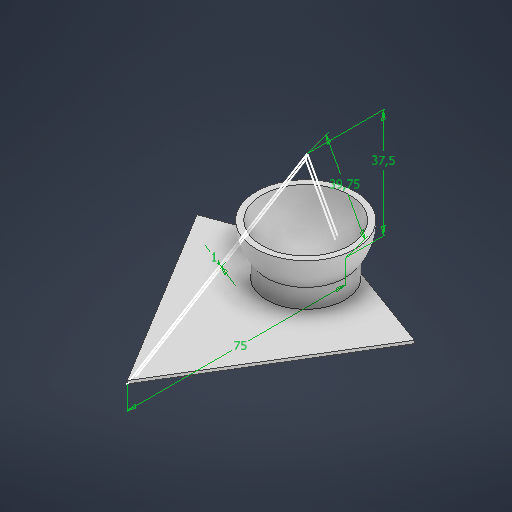
# Autodesk Inventor part: cabeza_1
Saved by Autodesk Inventor 2026.2 (Build 302298000, 298)
## iProperties
Created: 2026-05-21
Part Number: cabeza_1
Material: Generic
Document SubType Name: Modeling
Designer: juand
Density: 1 g/cm^3
Appearance: Default
Author: juand
Autodesk Inventor part; units mm, degrees
ref_plane "YZ Plane" through (0, 0, 0) normal (1, 0, 0) x (0, 1, 0)
ref_plane "XZ Plane" through (0, 0, 0) normal (0, 1, 0) x (-1, 0, 0)
ref_plane "XY Plane" through (0, 0, 0) normal (0, 0, 1) x (1, 0, 0)
sketch "Sketch1" plane through (0, 0, 0) normal (1, 0, 0) x (0, 1, 0)
  line L0 (0, 0) -> (0, 75)
  line L1 (0, 0) -> (37.5, 13.1838)
  line L2 (37.5, 13.1838) -> (0, 75)
  line L3 (0, 73.072) -> (36.006, 13.7185)
  line L4 (36.006, 13.7185) -> (0, 1.06)
  line L5 (36.006, 13.7185) -> (37.5, 13.1838)
  dimension "d0" = 75
  dimension "d1" = 37.5
  dimension "d2" = 39.75
  dimension "d3" = 1
  constraints: 12 end point, 2 point on line, 1 vertical, 1 other
  measures "d0" distance of L0.start L0.end
  measures "d1" horizontal distance of L1.end L0.start
  measures "d2" distance of L0.start L1.end
  measures "d3" distance between parallel lines of L2 L3
sketch "Sketch2" plane through (0, 0, 0) normal (0, 1, 0) x (-1, 0, 0)
  line L0 (0, 0) -> (-37.3077, 13.7185)
  line L1 (-37.3077, 13.7185) -> (0, 75)
  line L2 (0, 0) -> (0, 75) projected
  line L3 (0, 13.7185) -> (0, 1.06) projected
  line L4 (0, 13.7185) -> (-37.3077, 13.7185) construction
  line L5 (0, 1.0655) -> (-35.8211, 14.2374)
  line L6 (-35.8211, 14.2374) -> (0, 73.077)
  line L7 (0, 0) -> (37.3077, 13.7185)
  line L8 (37.3077, 13.7185) -> (0, 75)
  line L9 (0, 1.0655) -> (35.8211, 14.2374)
  line L10 (35.8211, 14.2374) -> (0, 73.077)
  line L11 (-35.8211, 14.2374) -> (-37.3077, 13.7185)
  line L12 (35.8211, 14.2374) -> (37.3077, 13.7185)
  dimension "d4" = 39.75
  dimension "d5" = 1
  constraints: 22 end point, 2 point on line, 2 symmetric about line, 1 perpendicular, 1 other
  measures "d4" distance of L0.start L0.end
  measures "d5" distance between parallel lines of L0 L5
extrude "Extrusion1" add sketch "Sketch2" along normal blind 1
sketch "Sketch6" plane through (0, 0, 0) normal (1, 0, 0) x (0, 1, 0)
  line L0 (37.5, 13.1838) -> (0, 75) projected
  line L1 (0, 73.072) -> (36.006, 13.7185) projected
  line L2 (0, 0) -> (37.5, 13.1838) projected
  line L3 (36.006, 13.7185) -> (0, 1.06) projected
  line L4 (1, 75) -> (1, 13.7185) projected
  line L5 (1, 13.7185) -> (1, 0) projected
  line L6 (36.006, 13.7185) -> (1, 13.7185)
  arc A0 (3, 13.7185) -> (18, -1.2815) centre (18, 13.7185) ccw
  line L7 (18, 13.7185) -> (18, -1.2815)
  line L8 (18, -1.2815) -> (18, -3.2815)
  arc A1 (1, 13.7185) -> (18, -3.2815) centre (18, 13.7185) ccw
  line L9 (1, 0.3516) -> (7.4965, 0.3516)
  dimension "d31" = 15
  dimension "d32" = 2
  constraints: 8 end point, 7 point on line, 5 point on circle, 2 centre point, 2 vertical, 1 coincident, 1 horizontal, 1 perpendicular
  measures "d31" radius of A0
  measures "d32" radial gap between concentric circles of A0 A1
revolve "Revolution4" add sketch "Sketch6" angle 360 about axis through (0, 36.006, 13.7185) along (0, -1, 0) contours A0 L8 A1 L2 | L2 A1 L3 A0 | A1 L3 L5 | L6 A0 L3 A1 | A1 L9 L2 | L2 L5 L3 A1
body "Solid7"
